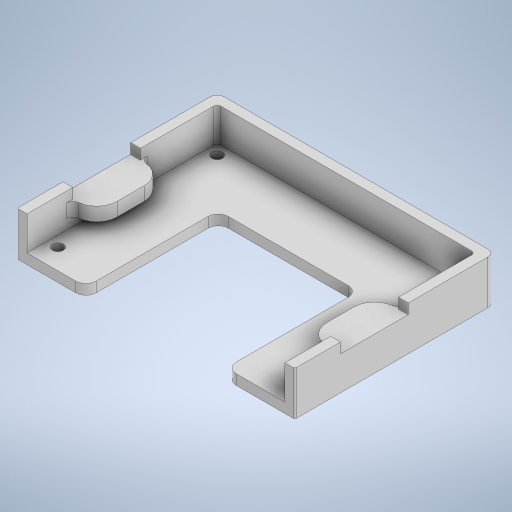
# Autodesk Inventor part: podstawa_PCB
Saved by Autodesk Inventor 2023 (Build 270158000, 158)
## iProperties
Created: 2024-04-28
Part Number: podstawa_PCB
Material: Ogólny
Document SubType Name: Modeling
Designer: kamil
Density: 1 g/cm^3
Appearance: Domyślna
Author: kamil
Autodesk Inventor part; units mm, degrees
ref_plane "YZ Plane" through (0, 0, 0) normal (1, 0, 0) x (0, 1, 0)
ref_plane "XZ Plane" through (0, 0, 0) normal (0, 1, 0) x (-1, 0, 0)
ref_plane "XY Plane" through (0, 0, 0) normal (0, 0, 1) x (1, 0, 0)
sketch "Szkic1" plane through (0, 0, 0) normal (0, 1, 0) x (-1, 0, 0)
  line L0 (41, 29.5365) -> (-41, 29.5365)
  line L1 (-41, 29.5365) -> (-41, -29.5365)
  line L2 (-41, -29.5365) -> (41, -29.5365)
  line L3 (41, -29.5365) -> (41, 29.5365)
  point P0 (0, 0)
  point P1 (-41, 0)
  point P2 (0, 29.5365)
  dimension "d0" = 82
  dimension "d1" = 59.073
  constraints: 8 end point, 2 midpoint, 2 parallel, 1 horizontal, 1 horizontal alignment, 1 perpendicular, 1 vertical alignment
  measures "d0" distance of L0.start L0.end
  measures "d1" distance of L0.end L1.end
extrude "Wyciągnięcie proste1" add sketch "Szkic1" along normal blind 3
sketch "Szkic2" plane through (0, 3, 0) normal (0, 1, 0) x (1, 0, 0)
  circle A0 centre (-35, -23.5365) radius 6
  circle A1 centre (35, -23.5365) radius 6
  circle A2 centre (35, 23.5365) radius 6
  circle A3 centre (-35, 23.5365) radius 6
  line L0 (-41, 29.5365) -> (-41, -29.5365) projected
  line L1 (-41, -29.5365) -> (41, -29.5365) projected
  line L2 (41, -29.5365) -> (41, 29.5365) projected
  line L3 (41, 29.5365) -> (-41, 29.5365) projected
  point P0 (0, 0)
  dimension "d4" = 12
  dimension "d5" = 12
  dimension "d6" = 12
  dimension "d7" = 12
  constraints: 8 tangent, 4 centre point, 4 coincident
  measures "d4" diameter of A0
  measures "d5" diameter of A1
  measures "d6" diameter of A2
  measures "d7" diameter of A3
hole "Otwór1" at (35, 3, 23.5365) at (35, 3, -23.5365) at (-35, 3, -23.5365) at (-35, 3, 23.5365) direction (0, -1, 0) diameter 3.2 end through all
fillet "Zaokrąglenie1" radius 2 2 edges at (-41, 1.5, -29.5365) (41, 1.5, -29.5365)
sketch "Szkic3" plane through (0, 3, 0) normal (0, 1, 0) x (1, 0, 0)
  line L0 (-41, 27.5365) -> (-41, -29.5365) projected
  arc A0 (-39, 29.5365) -> (-41, 27.5365) centre (-39, 27.5365) ccw projected
  line L1 (39, 29.5365) -> (-39, 29.5365) projected
  arc A1 (41, 27.5365) -> (39, 29.5365) centre (39, 27.5365) ccw projected
  line L2 (41, -29.5365) -> (41, 27.5365) projected
  line L3 (-38.1, -29.5365) -> (-38.1, 26.6365)
  line L4 (-38.1, 26.6365) -> (38.1, 26.6365)
  line L5 (38.1, 26.6365) -> (38.1, -29.5365)
  line L6 (-41, -29.5365) -> (41, -29.5365) projected
  point P0 (0, 0)
  dimension "d16" = 2.9
  constraints: 6 end point, 2 other
  measures "d16" distance between parallel lines of L0 L3
extrude "Wyciągnięcie proste2" add sketch "Szkic3" along normal blind 3 contours A0 L1 A1 L2 L6 L5 L4 L3 L0
sketch "Szkic4" plane through (0, 6, 0) normal (0, 1, 0) x (1, 0, 0)
  line L0 (-41, -29.5365) -> (-38.1, -29.5365) projected
  line L1 (-38.1, -29.5365) -> (-38.1, 26.6365) projected
  line L2 (-38.1, 26.6365) -> (38.1, 26.6365) projected
  line L3 (38.1, 26.6365) -> (38.1, -29.5365) projected
  line L4 (38.1, -29.5365) -> (41, -29.5365) projected
  line L5 (41, -29.5365) -> (41, 27.5365) projected
  arc A0 (41, 27.5365) -> (39, 29.5365) centre (39, 27.5365) ccw projected
  line L6 (39, 29.5365) -> (-39, 29.5365) projected
  arc A1 (-39, 29.5365) -> (-41, 27.5365) centre (-39, 27.5365) ccw projected
  line L7 (-41, 27.5365) -> (-41, -29.5365) projected
  circle A2 centre (-35, 23.5365) radius 1.6 projected
  circle A3 centre (-35, -23.5365) radius 1.6 projected
  circle A4 centre (35, -23.5365) radius 1.6 projected
  circle A5 centre (-35, -23.5365) radius 7.5
  circle A6 centre (-35, 23.5365) radius 1.6 projected
  circle A7 centre (-35, 23.5365) radius 7.5
  circle A8 centre (35, 23.5365) radius 1.6 projected
  circle A9 centre (35, -23.5365) radius 7.5
  circle A10 centre (35, 23.5365) radius 7.5
  line L8 (39, 29.5365) -> (-39, 29.5365) projected
  line L9 (-27.5, 29.5365) -> (27.5, 29.5365)
  line L10 (27.5, 29.5365) -> (27.5, 19.5365)
  line L11 (27.5, 19.5365) -> (-27.5, 19.5365)
  line L12 (-27.5, 19.5365) -> (-27.5, 29.5365)
  line L13 (-41, 27.5365) -> (-41, -29.5365) projected
  line L14 (-41, 3.9635) -> (-31, 3.9635)
  line L15 (-31, 3.9635) -> (-31, -16.0365)
  line L16 (-31, -16.0365) -> (-41, -16.0365)
  line L17 (-41, -16.0365) -> (-41, 3.9635)
  line L18 (41, -29.5365) -> (41, 27.5365) projected
  line L19 (41, 3.9635) -> (31, 3.9635)
  line L20 (31, 3.9635) -> (31, -16.0365)
  line L21 (31, -16.0365) -> (41, -16.0365)
  line L22 (41, -16.0365) -> (41, 3.9635)
  point P0 (0, 0)
  point P1 (-38.1, 3.9635)
  point P2 (-27.5, 26.6365)
  point P3 (27.5, 26.6365)
  point P4 (38.1, 3.9635)
  point P5 (38.1, -16.0365)
  point P6 (-38.1, -16.0365)
  point P7 (40.8967, 28.1711)
  point P8 (39.6346, 29.4332)
  dimension "d19" = 15
  dimension "d20" = 15
  dimension "d21" = 15
  dimension "d22" = 15
  dimension "d23" = 10
  dimension "d24" = 10
  dimension "d25" = 10
  dimension "d49" = 20
  dimension "d50" = 20
  constraints: 24 end point, 6 parallel, 4 centre point, 4 coincident, 4 tangent, 3 horizontal, 3 perpendicular, 3 point on line
  measures "d19" diameter of A5
  measures "d20" diameter of A7
  measures "d21" diameter of A9
  measures "d22" diameter of A10
  measures "d23" distance of L9.end L10.end
  measures "d24" distance of L14.start L14.end
  measures "d25" distance of L21.end L20.end
  measures "d49" distance between parallel lines of L16 L14
  measures "d50" distance between parallel lines of L21 L19
extrude "Wyciągnięcie proste3" add sketch "Szkic4" along normal blind 4 contours L7 A5 L0 | A5 L7 L1 L0 | L7 L16 L1 A5 | L16 L1 L14 L15 | L7 L14 L1 L16 | L7 A7 L1 L14 | L7 A1 A7 L6 L2 L1 | A1 A7 | A7 L6 L12 L2 | L12 L6 L10 L2 | L10 L6 A10 L2 | A10 L6 A0 L5 L3 L2 | A10 L5 L19 L3 | L19 L5 L21 L3 | L3 L21 L20 L19 | A0 A10 | L21 L5 A9 L3 | A9 L5 L4 L3 | A9 L5 L4
fillet "Zaokrąglenie3" radius 1 2 edges at (38.1, 6.5, -26.6365) (-38.1, 6.5, -26.6365)
sketch "Szkic6" plane through (0, 3, 0) normal (0, 1, 0) x (1, 0, 0)
  line L0 (-20.7, 9.5365) -> (20.7, 9.5365)
  line L1 (20.7, 9.5365) -> (20.7, -29.5365)
  line L2 (20.7, -29.5365) -> (-20.7, -29.5365)
  line L3 (-20.7, -29.5365) -> (-20.7, 9.5365)
  line L4 (-38.1, -29.5365) -> (38.1, -29.5365) projected
  point P0 (0, 0)
  point P1 (0, -29.5365)
  point P2 (0, -29.5365)
  point P3 (0, -29.5365)
  dimension "d33" = 39.073
  dimension "d34" = 41.4
  constraints: 8 end point, 3 midpoint, 2 coincident, 2 parallel, 1 horizontal, 1 perpendicular
  measures "d33" distance of L0.end L1.end
  measures "d34" distance of L1.end L2.end
extrude "Wyciągnięcie proste5" cut sketch "Szkic6" against normal up to surface (3 mm away)
fillet "Zaokrąglenie5" radius 3 4 edges at (-20.7, 1.5, -9.5365) (20.7, 1.5, -9.5365) (20.7, 1.5, 29.5365) (-20.7, 1.5, 29.5365)
sketch "Szkic8" plane through (0, 10, 0) normal (0, 1, 0) x (1, 0, 0)
  line L0 (-38.1, 3.9635) -> (-38.1, 25.6365) projected
  arc A0 (-37.1, 26.6365) -> (-38.1, 25.6365) centre (-37.1, 25.6365) ccw projected
  line L1 (-37.1, 26.6365) -> (37.1, 26.6365) projected
  arc A1 (38.1, 25.6365) -> (37.1, 26.6365) centre (37.1, 25.6365) ccw projected
  line L2 (38.1, 25.6365) -> (38.1, 3.9635) projected
  line L3 (38.1, -16.0365) -> (38.1, -29.5365) projected
  line L4 (38.1, -29.5365) -> (41, -29.5365) projected
  line L5 (41, -29.5365) -> (41, 27.5365) projected
  arc A2 (41, 27.5365) -> (39, 29.5365) centre (39, 27.5365) ccw projected
  line L6 (39, 29.5365) -> (-39, 29.5365) projected
  arc A3 (-39, 29.5365) -> (-41, 27.5365) centre (-39, 27.5365) ccw projected
  line L7 (-41, 27.5365) -> (-41, -29.5365) projected
  line L8 (-41, -29.5365) -> (-38.1, -29.5365) projected
  line L9 (-38.1, -29.5365) -> (-38.1, -16.0365) projected
  line L10 (-31, 3.9635) -> (-38.1, 3.9635) projected
  line L11 (-38.1, 3.9635) -> (-41, 3.9635)
  line L12 (-38.1, -16.0365) -> (-38.1, 3.9635) projected
  line L13 (-38.1, -16.0365) -> (-41, -16.0365)
  line L14 (38.1, 3.9635) -> (41, 3.9635)
  line L15 (38.1, -16.0365) -> (41, -16.0365)
  line L16 (38.1, 3.9635) -> (31, 3.9635) projected
  line L17 (31, 3.9635) -> (31, -16.0365) projected
  line L18 (31, -16.0365) -> (38.1, -16.0365) projected
  line L19 (-38.1, -16.0365) -> (-31, -16.0365) projected
  line L20 (-31, -16.0365) -> (-31, 3.9635) projected
  line L21 (-31, 3.9635) -> (-38.1, 3.9635) projected
  point P0 (0, 0)
  point P1 (-37, 16.0365)
  constraints: 8 end point, 6 point on line, 1 parallel, 1 perpendicular, 1 other
extrude "Wyciągnięcie proste7" add sketch "Szkic8" along normal blind 3 contours L11 L7 A3 L6 A2 L5 L14 L2 A1 L1 A0 L0 | L9 L8 L7 L13 | L5 L4 L3 L15
fillet "Zaokrąglenie8" radius 0.5 2 edges at (-41, 6.5, 29.5365) (41, 6.5, 29.5365)
sketch "Szkic9" plane through (39, 0, -29.5365) normal (0, 0, -1) x (-1, 0, 0)
  line L0 (0, 0) -> (0, 13) projected
  line L1 (0, 0) -> (78, 0) projected
  line L2 (78, 13) -> (78, 0) projected
  line L3 (0, 13) -> (78, 13) projected
  line L4 (0, 13) -> (78, 13) construction
  line L5 (78, 13) -> (78, 0) construction
  line L6 (78, 0) -> (0, 0) construction
  line L7 (0, 0) -> (0, 13) construction
  line L8 (18.0857, 2.9257) -> (16.2914, 2.9257)
  line L9 (16.2914, 2.9257) -> (16.2914, 7.6114)
  line L10 (16.2914, 7.6114) -> (14.9943, 4.5714)
  line L11 (14.9943, 4.5714) -> (13.7429, 4.5714)
  line L12 (13.7429, 4.5714) -> (12.4457, 7.6114)
  line L13 (12.4457, 7.6114) -> (12.4457, 2.9257)
  line L14 (12.4457, 2.9257) -> (10.7429, 2.9257)
  line L15 (10.7429, 2.9257) -> (10.7429, 9.9257)
  line L16 (10.7429, 9.9257) -> (12.84, 9.9257)
  line L17 (12.84, 9.9257) -> (14.4171, 6.4114)
  line L18 (14.4171, 6.4114) -> (15.9886, 9.9257)
  line L19 (15.9886, 9.9257) -> (18.0857, 9.9257)
  line L20 (18.0857, 9.9257) -> (18.0857, 2.9257)
  spline S0 degree 2 poles (25.1771, 5.5657) (25.1771, 4.2629) (23.6571, 2.76) (22.2857, 2.76) knots 0 0 0 1 2 2 2
  spline S1 degree 2 poles (22.2857, 2.76) (20.9086, 2.76) (19.3886, 4.2629) (19.3886, 5.5657) knots 0 0 0 1 2 2 2
  spline S2 degree 2 poles (19.3886, 5.5657) (19.3886, 6.8743) (20.92, 8.3714) (22.2857, 8.3714) knots 0 0 0 1 2 2 2
  spline S3 degree 2 poles (22.2857, 8.3714) (23.6686, 8.3714) (25.1771, 6.8686) (25.1771, 5.5657) knots 0 0 0 1 2 2 2
  spline S4 degree 2 poles (23.0914, 4.28) (23.2571, 4.4857) (23.4229, 5.0514) (23.4229, 5.5543) knots 0 0 0 1 2 2 2
  spline S5 degree 2 poles (23.4229, 5.5543) (23.4229, 6.0171) (23.2514, 6.6457) (23.1029, 6.8343) knots 0 0 0 1 2 2 2
  spline S6 degree 2 poles (23.1029, 6.8343) (22.9543, 7.0286) (22.5257, 7.1886) (22.2857, 7.1886) knots 0 0 0 1 2 2 2
  spline S7 degree 2 poles (22.2857, 7.1886) (22.04, 7.1886) (21.6571, 7.0571) (21.48, 6.8571) knots 0 0 0 1 2 2 2
  spline S8 degree 2 poles (21.48, 6.8571) (21.3257, 6.6743) (21.1429, 6.04) (21.1429, 5.5543) knots 0 0 0 1 2 2 2
  spline S9 degree 2 poles (21.1429, 5.5543) (21.1429, 5.12) (21.3029, 4.4857) (21.4571, 4.2971) knots 0 0 0 1 2 2 2
  spline S10 degree 2 poles (21.4571, 4.2971) (21.6114, 4.1143) (22.0286, 3.9429) (22.2971, 3.9429) knots 0 0 0 1 2 2 2
  spline S11 degree 2 poles (22.2971, 3.9429) (22.5257, 3.9429) (22.9486, 4.0971) (23.0914, 4.28) knots 0 0 0 1 2 2 2
  line L21 (31.52, 2.9257) -> (29.8229, 2.9257)
  line L22 (29.8229, 2.9257) -> (29.8229, 3.4743)
  spline S12 degree 2 poles (29.8229, 3.4743) (29.3886, 3.12) (28.6286, 2.7771) (28.1257, 2.7771) knots 0 0 0 1 2 2 2
  spline S13 degree 2 poles (28.1257, 2.7771) (27.1657, 2.7771) (26.0114, 4.2629) (26.0114, 5.5257) knots 0 0 0 1 2 2 2
  spline S14 degree 2 poles (26.0114, 5.5257) (26.0114, 6.1943) (26.4, 7.2343) (26.7371, 7.6057) knots 0 0 0 1 2 2 2
  spline S15 degree 2 poles (26.7371, 7.6057) (27.0571, 7.96) (27.9714, 8.3486) (28.4229, 8.3486) knots 0 0 0 1 2 2 2
  spline S16 degree 2 poles (28.4229, 8.3486) (28.8971, 8.3486) (29.5029, 8.1486) (29.8229, 7.9886) knots 0 0 0 1 2 2 2
  line L23 (29.8229, 7.9886) -> (29.8229, 10.24)
  line L24 (29.8229, 10.24) -> (31.52, 10.24)
  line L25 (31.52, 10.24) -> (31.52, 2.9257)
  line L26 (29.8229, 4.3771) -> (29.8229, 6.9714)
  spline S17 degree 2 poles (29.8229, 6.9714) (29.6457, 7.0457) (29.2514, 7.1143) (29.0857, 7.1143) knots 0 0 0 1 2 2 2
  spline S18 degree 2 poles (29.0857, 7.1143) (28.4229, 7.1143) (27.7543, 6.28) (27.7543, 5.5429) knots 0 0 0 1 2 2 2
  spline S19 degree 2 poles (27.7543, 5.5429) (27.7543, 4.7657) (28.2914, 4.0629) (28.88, 4.0629) knots 0 0 0 1 2 2 2
  spline S20 degree 2 poles (28.88, 4.0629) (29.1086, 4.0629) (29.6286, 4.2343) (29.8229, 4.3771) knots 0 0 0 1 2 2 2
  spline S21 degree 2 poles (39.2057, 5.0686) (39.2057, 4.56) (38.7943, 3.76) (38.44, 3.4971) knots 0 0 0 1 2 2 2
  spline S22 degree 2 poles (38.44, 3.4971) (38.0229, 3.1886) (37.0343, 2.9257) (36.2686, 2.9257) knots 0 0 0 1 2 2 2
  line L27 (36.2686, 2.9257) -> (33.2114, 2.9257)
  line L28 (33.2114, 2.9257) -> (33.2114, 9.9257)
  line L29 (33.2114, 9.9257) -> (35.9314, 9.9257)
  spline S23 degree 2 poles (35.9314, 9.9257) (36.7771, 9.9257) (37.56, 9.8114) (37.9486, 9.6229) knots 0 0 0 1 2 2 2
  spline S24 degree 2 poles (37.9486, 9.6229) (38.3486, 9.4171) (38.7371, 8.7371) (38.7371, 8.2971) knots 0 0 0 1 2 2 2
  spline S25 degree 2 poles (38.7371, 8.2971) (38.7371, 7.7886) (38.2, 7.0171) (37.7086, 6.8) knots 0 0 0 1 2 2 2
  line L30 (37.7086, 6.8) -> (37.7086, 6.76)
  spline S26 degree 2 poles (37.7086, 6.76) (38.4, 6.6229) (39.2057, 5.7714) (39.2057, 5.0686) knots 0 0 0 1 2 2 2
  spline S27 degree 2 poles (37.3314, 5.0971) (37.3314, 5.4343) (37.0743, 5.7943) (36.76, 5.8857) knots 0 0 0 1 2 2 2
  spline S28 degree 2 poles (36.76, 5.8857) (36.5486, 5.9429) (35.8057, 5.9543) (35.4, 5.9543) knots 0 0 0 1 2 2 2
  line L31 (35.4, 5.9543) -> (35.0057, 5.9543)
  line L32 (35.0057, 5.9543) -> (35.0057, 4.2114)
  line L33 (35.0057, 4.2114) -> (35.1371, 4.2114)
  spline S29 degree 2 poles (35.1371, 4.2114) (35.9029, 4.2114) (36.56, 4.2229) (36.8343, 4.3371) knots 0 0 0 1 2 2 2
  spline S30 degree 2 poles (36.8343, 4.3371) (37.12, 4.4571) (37.3314, 4.8457) (37.3314, 5.0971) knots 0 0 0 1 2 2 2
  spline S31 degree 2 poles (36.8914, 7.9429) (36.8914, 8.12) (36.7143, 8.4686) (36.4971, 8.5486) knots 0 0 0 1 2 2 2
  spline S32 degree 2 poles (36.4971, 8.5486) (36.2971, 8.6286) (35.7086, 8.64) (35.1771, 8.64) knots 0 0 0 1 2 2 2
  line L34 (35.1771, 8.64) -> (35.0057, 8.64)
  line L35 (35.0057, 8.64) -> (35.0057, 7.16)
  line L36 (35.0057, 7.16) -> (35.2914, 7.16)
  spline S33 degree 2 poles (35.2914, 7.16) (35.72, 7.16) (36.32, 7.1886) (36.4971, 7.2686) knots 0 0 0 1 2 2 2
  spline S34 degree 2 poles (36.4971, 7.2686) (36.7429, 7.3771) (36.8914, 7.72) (36.8914, 7.9429) knots 0 0 0 1 2 2 2
  spline S35 degree 2 poles (45.8571, 5.5657) (45.8571, 4.2629) (44.3371, 2.76) (42.9657, 2.76) knots 0 0 0 1 2 2 2
  spline S36 degree 2 poles (42.9657, 2.76) (41.5886, 2.76) (40.0686, 4.2629) (40.0686, 5.5657) knots 0 0 0 1 2 2 2
  spline S37 degree 2 poles (40.0686, 5.5657) (40.0686, 6.8743) (41.6, 8.3714) (42.9657, 8.3714) knots 0 0 0 1 2 2 2
  spline S38 degree 2 poles (42.9657, 8.3714) (44.3486, 8.3714) (45.8571, 6.8686) (45.8571, 5.5657) knots 0 0 0 1 2 2 2
  spline S39 degree 2 poles (43.7714, 4.28) (43.9371, 4.4857) (44.1029, 5.0514) (44.1029, 5.5543) knots 0 0 0 1 2 2 2
  spline S40 degree 2 poles (44.1029, 5.5543) (44.1029, 6.0171) (43.9314, 6.6457) (43.7829, 6.8343) knots 0 0 0 1 2 2 2
  spline S41 degree 2 poles (43.7829, 6.8343) (43.6343, 7.0286) (43.2057, 7.1886) (42.9657, 7.1886) knots 0 0 0 1 2 2 2
  spline S42 degree 2 poles (42.9657, 7.1886) (42.72, 7.1886) (42.3371, 7.0571) (42.16, 6.8571) knots 0 0 0 1 2 2 2
  spline S43 degree 2 poles (42.16, 6.8571) (42.0057, 6.6743) (41.8229, 6.04) (41.8229, 5.5543) knots 0 0 0 1 2 2 2
  spline S44 degree 2 poles (41.8229, 5.5543) (41.8229, 5.12) (41.9829, 4.4857) (42.1371, 4.2971) knots 0 0 0 1 2 2 2
  spline S45 degree 2 poles (42.1371, 4.2971) (42.2914, 4.1143) (42.7086, 3.9429) (42.9771, 3.9429) knots 0 0 0 1 2 2 2
  spline S46 degree 2 poles (42.9771, 3.9429) (43.2057, 3.9429) (43.6286, 4.0971) (43.7714, 4.28) knots 0 0 0 1 2 2 2
  spline S47 degree 2 poles (50.4457, 2.9714) (50.1714, 2.9029) (49.56, 2.8229) (49.12, 2.8229) knots 0 0 0 1 2 2 2
  spline S48 degree 2 poles (49.12, 2.8229) (48.1314, 2.8229) (47.1657, 3.6229) (47.1657, 4.5886) knots 0 0 0 1 2 2 2
  line L37 (47.1657, 4.5886) -> (47.1657, 7.0571)
  line L38 (47.1657, 7.0571) -> (46.4686, 7.0571)
  line L39 (46.4686, 7.0571) -> (46.4686, 8.2057)
  line L40 (46.4686, 8.2057) -> (47.1657, 8.2057)
  line L41 (47.1657, 8.2057) -> (47.1657, 9.7143)
  line L42 (47.1657, 9.7143) -> (48.8629, 9.7143)
  line L43 (48.8629, 9.7143) -> (48.8629, 8.2057)
  line L44 (48.8629, 8.2057) -> (50.4457, 8.2057)
  line L45 (50.4457, 8.2057) -> (50.4457, 7.0571)
  line L46 (50.4457, 7.0571) -> (48.8629, 7.0571)
  line L47 (48.8629, 7.0571) -> (48.8629, 5.1829)
  spline S49 degree 2 poles (48.8629, 5.1829) (48.8629, 4.9086) (48.8743, 4.4914) (48.9429, 4.3314) knots 0 0 0 1 2 2 2
  spline S50 degree 2 poles (48.9429, 4.3314) (49.0057, 4.1657) (49.3429, 3.9714) (49.6629, 3.9714) knots 0 0 0 1 2 2 2
  spline S51 degree 2 poles (49.6629, 3.9714) (49.7943, 3.9714) (50.2229, 4.0857) (50.3029, 4.1314) knots 0 0 0 1 2 2 2
  line L48 (50.3029, 4.1314) -> (50.4457, 4.1314)
  line L49 (50.4457, 4.1314) -> (50.4457, 2.9714)
  line L50 (61.1886, 9.9257) -> (58.6343, 2.9257)
  line L51 (58.6343, 2.9257) -> (56.6171, 2.9257)
  line L52 (56.6171, 2.9257) -> (54.0629, 9.9257)
  line L53 (54.0629, 9.9257) -> (55.9543, 9.9257)
  line L54 (55.9543, 9.9257) -> (57.6457, 5.0114)
  line L55 (57.6457, 5.0114) -> (59.3371, 9.9257)
  line L56 (59.3371, 9.9257) -> (61.1886, 9.9257)
  line L57 (67.2286, 2.9257) -> (62.5543, 2.9257)
  line L58 (62.5543, 2.9257) -> (62.5543, 4.1486)
  line L59 (62.5543, 4.1486) -> (64.0286, 4.1486)
  line L60 (64.0286, 4.1486) -> (64.0286, 7.8457)
  line L61 (64.0286, 7.8457) -> (62.5543, 7.8457)
  line L62 (62.5543, 7.8457) -> (62.5543, 8.9886)
  spline S52 degree 2 poles (62.5543, 8.9886) (62.8914, 8.9886) (63.5143, 9.0686) (63.72, 9.1657) knots 0 0 0 1 2 2 2
  spline S53 degree 2 poles (63.72, 9.1657) (63.9657, 9.2857) (64.2057, 9.6629) (64.2286, 9.9429) knots 0 0 0 1 2 2 2
  line L63 (64.2286, 9.9429) -> (65.7829, 9.9429)
  line L64 (65.7829, 9.9429) -> (65.7829, 4.1486)
  line L65 (65.7829, 4.1486) -> (67.2286, 4.1486)
  line L66 (67.2286, 4.1486) -> (67.2286, 2.9257)
  point P0 (39, 0)
  point P1 (0, 6.5)
  point P2 (0, 6.5)
  point P3 (39, 0)
  point P4 (39, 0)
  dimension "d45" = 13
  dimension "d46" = 78
  constraints: 4 midpoint, 2 coincident, 2 other
  measures "d45" distance of L6.end L4.start
  measures "d46" distance of L5.end L6.end
extrude "Wyciągnięcie proste8" cut sketch "Szkic9" against normal blind 1 contours L8 L9 L10 L11 L12 L13 L14 L15 L16 L17 L18 L19 L20 | S0 S1 S2 S3 | L21 L22 S12 S13 S14 S15 S16 L23 L24 L25 | S21 S22 L27 L28 L29 S23 S24 S25 L30 S26 | S35 S36 S37 S38 | S47 S48 L37 L38 L39 L40 L41 L42 L43 L44 L45 L46 L47 S49 S50 S51 L48 L49 | L50 L51 L52 L53 L54 L55 L56 | L57 L58 L59 L60 L61 L62 S52 S53 L63 L64 L65 L66
fillet "Zaokrąglenie9" radius 6 4 edges at (-31, 8, -3.9635) (-31, 8, 16.0365) (31, 8, -3.9635) (31, 8, 16.0365)
fillet "Zaokrąglenie10" radius 2 4 edges at (-38.1, 8, 16.0365) (-38.1, 8, -3.9635) (38.1, 8, -3.9635) (38.1, 8, 16.0365)
